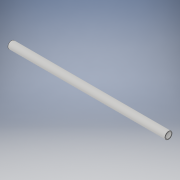
# Autodesk Inventor part: PVC Pipe 1.25 IN D
Saved by Autodesk Inventor 2019 (Build 230136000, 136)
## iProperties
Created: 2019-07-05
Part Number: PVC Pipe 1.25 IN D
Material: Generic
Document SubType Name: Modeling
Designer: J. LENDI
Mass: 419.78 g
Surface Area: 2212.75 cm^2
Volume: 419.78 cm^3
Density: 1 g/cm^3
Appearance: Default
Author: J. LENDI
Autodesk Inventor part; units mm, degrees
ref_plane "YZ Plane" through (0, 0, 0) normal (1, 0, 0) x (0, 1, 0)
ref_plane "XZ Plane" through (0, 0, 0) normal (0, 1, 0) x (-1, 0, 0)
ref_plane "XY Plane" through (0, 0, 0) normal (0, 0, 1) x (1, 0, 0)
sketch "Sketch1" plane through (0, 0, 0) normal (1, 0, 0) x (0, 1, 0)
  circle A0 centre (0, 0) radius 21.082
  circle A1 centre (0, 0) radius 17.272
  dimension "d0" = 42.164
  dimension "d1" = 34.544
  constraints: 2 centre point, 2 coincident
  measures "d0" diameter of A0
  measures "d1" diameter of A1
extrude "Extrusion1" add sketch "Sketch1" along normal mid plane 914.4
body "Solid1"
